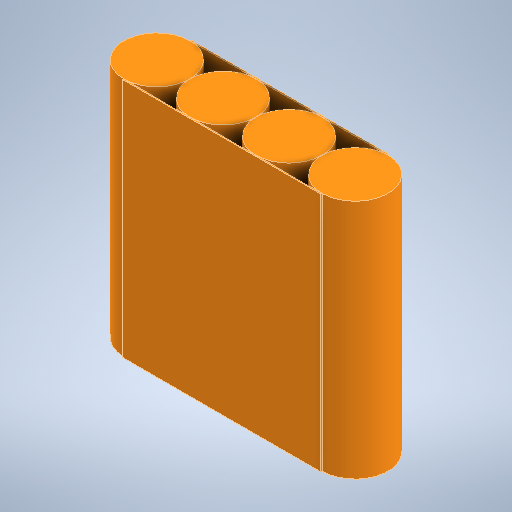
# Autodesk Inventor part: NiMH-Battery
Saved by Autodesk Inventor 2025.3 (Build 293356000, 356)
## iProperties
Created: 2025-06-02
Part Number: NiMH-Battery
Material: 一般
Document SubType Name: Modeling
Designer: yamashita1
Density: 1 g/cm^3
Appearance: オレンジ
Author: yamashita1
Autodesk Inventor part; units mm, degrees
ref_plane "YZ Plane" through (0, 0, 0) normal (1, 0, 0) x (0, 1, 0)
ref_plane "XZ Plane" through (0, 0, 0) normal (0, 1, 0) x (-1, 0, 0)
sketch "スケッチ1" plane through (0, 0, 0) normal (0, 1, 0) x (-1, 0, 0)
  circle A0 centre (21, 0) radius 7
  circle A1 centre (7, 0) radius 7
  circle A2 centre (-7, 0) radius 7
  circle A3 centre (-21, 0) radius 7
  line L0 (37.3253, 0) -> (-37.3253, 0) construction
  line L1 (0, 20.4736) -> (0, -20.4736) construction
  point P0 (0, 0)
  point P1 (0, 0)
  point P2 (-14, 0)
  point P3 (0, 0)
  point P4 (14, 0)
  dimension "d0" = 14
  dimension "d1" = 14
  dimension "d2" = 14
  dimension "d3" = 14
  constraints: 4 centre point, 4 end point, 4 point on line, 3 equal radius, 2 midpoint, 1 coincident, 1 horizontal, 1 symmetric about line, 1 vertical
  measures "d0" diameter of A0
  measures "d1" distance of A1.centre A0.centre
  measures "d2" distance of A2.centre A1.centre
  measures "d3" distance of A3.centre A2.centre
extrude "押し出し1" add sketch "スケッチ1" along normal blind 51
ref_plane "作業平面1" through (0, 0, 7) normal (0, 0, 1) x (1, 0, 0)
sketch "スケッチ2" plane through (0, 0, 7) normal (0, 0, 1) x (1, 0, 0)
  line L0 (-21, 51) -> (21, 51)
  line L1 (21, 51) -> (21, 0)
  line L2 (21, 0) -> (-21, 0)
  line L3 (-21, 0) -> (-21, 51)
  point P0 (0, 0)
  point P1 (0, 0)
  dimension "d7" = 51
  dimension "d8" = 42
  constraints: 8 end point, 2 parallel, 1 coincident, 1 horizontal, 1 midpoint, 1 perpendicular
  measures "d7" distance of L0.end L1.end
  measures "d8" distance of L0.start L0.end
extrude "押し出し2" add sketch "スケッチ2" along normal blind 0.25
mirror "ミラー1" about plane through (0, 0, 0) normal (0, 0, 1) of "押し出し2"
equation "\"d1\" = d0"
equation "\"d2\" = d1"
equation "\"d3\" = d2"
equation "\"d7\" = d4"
equation "\"d8\" = 3 * d0"
equation "\"d6\" = 0.5 * d0"
equation "\"d4\" = 51"
